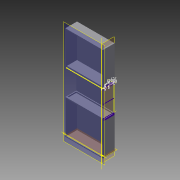
# Autodesk Inventor part: kontroller
Saved by Autodesk Inventor 2015 (Build 190159000, 159)
## iProperties
Created: 2015-12-13
Part Number: kontroller
Material: Generic
Document SubType Name: Modeling
Designer: abberik
Density: 1 g/cm^3
Appearance: Default
Author: abberik
Autodesk Inventor part; units mm, degrees
sketch "Sketch1" plane through (0, 0, 0) normal (0, 1, 0) x (-1, 0, 0)
  point P0 (0, 0)
sketch "Sketch2" plane through (0, 0, 0) normal (0, 1, 0) x (-1, 0, 0)
  point P0 (0, 0)
sketch "Sketch3" plane through (0, 0, 0) normal (0, 1, 0) x (-1, 0, 0)
  line L0 (93.3518, 235.1866) -> (-3.1482, 235.1866)
  line L1 (-3.1482, 235.1866) -> (-3.1482, -6.0634)
  line L2 (-3.1482, -6.0634) -> (93.3518, -6.0634)
  line L3 (93.3518, -6.0634) -> (93.3518, 235.1866)
  point P0 (0, 0)
  dimension "d0" = 241.25
  dimension "d1" = 96.5
  constraints: 8 end point, 2 parallel, 1 horizontal, 1 perpendicular
  measures "d0" distance of L2.end L0.start
  measures "d1" distance between parallel lines of L1 L3
extrude "Extrusion1" add sketch "Sketch3" along normal blind 30
sketch "Sketch4" plane through (0, 0, 0) normal (0, -1, 0) x (1, 0, 0)
  line L0 (-93.3518, -6.0634) -> (-93.3518, 235.1866) projected
  line L1 (-93.3518, 82.5616) -> (3.1482, 82.5616)
  line L2 (3.1482, 82.5616) -> (3.1482, 146.5616)
  line L3 (3.1482, 146.5616) -> (-93.3518, 146.5616)
  line L4 (-93.3518, 146.5616) -> (-93.3518, 82.5616)
  point P0 (0, 0)
  point P1 (-93.3518, 114.5616)
  point P2 (-93.3518, 114.5616)
  dimension "d4" = 64
  dimension "d5" = 0
  dimension "d6" = 96.5
  dimension "d7" = 0
  constraints: 8 end point, 2 midpoint, 2 parallel, 1 horizontal, 1 perpendicular
  measures "d4" distance between parallel lines of L3 L1
  measures "d5" distance of point (-93.352, 114.562) point (-93.352, 114.562)
  measures "d6" distance between parallel lines of L2 L4
  measures "d7" distance between parallel lines of L0 L4
extrude "Extrusion2" cut sketch "Sketch4" against normal blind 28
sketch "Sketch5" plane through (0, 0, 0) normal (0, -1, 0) x (1, 0, 0)
  line L0 (3.1482, 82.5616) -> (-93.3518, 82.5616) projected
  line L1 (-93.3518, -6.0634) -> (-93.3518, 82.5616) projected
  line L2 (3.1482, -6.0634) -> (-93.3518, -6.0634) projected
  line L3 (3.1482, 82.5616) -> (3.1482, -6.0634) projected
  line L4 (-93.3518, 146.5616) -> (3.1482, 146.5616) projected
  line L5 (3.1482, 235.1866) -> (3.1482, 146.5616) projected
  line L6 (-93.3518, 235.1866) -> (3.1482, 235.1866) projected
  line L7 (-93.3518, 146.5616) -> (-93.3518, 235.1866) projected
  line L8 (-91.3518, 80.5616) -> (1.1482, 80.5616)
  line L9 (1.1482, 80.5616) -> (1.1482, -4.0634)
  line L10 (1.1482, -4.0634) -> (-91.3518, -4.0634)
  line L11 (-91.3518, -4.0634) -> (-91.3518, 80.5616)
  line L12 (-91.3518, 233.1866) -> (1.1482, 233.1866)
  line L13 (1.1482, 233.1866) -> (1.1482, 148.5616)
  line L14 (1.1482, 148.5616) -> (-91.3518, 148.5616)
  line L15 (-91.3518, 148.5616) -> (-91.3518, 233.1866)
  point P0 (0, 0)
  dimension "d10" = 2
  dimension "d11" = 2
  constraints: 16 end point, 6 other
  measures "d10" distance between parallel lines of L1 L11
  measures "d11" distance between parallel lines of L7 L15
extrude "Extrusion3" cut sketch "Sketch5" against normal blind 28 contours L8 L9 L10 L11 | L12 L13 L14 L15
sketch "Sketch6" plane through (-93.3518, 0, 235.1866) normal (-1, 0, 0) x (0, 0, 1)
  point P0 (-235.1866, 0)
  point P1 (-196.9375, 14)
sketch "Sketch7" plane through (-91.3518, 0, 148.5616) normal (0, 0, 1) x (1, 0, 0)
  line L0 (92.5, 0) -> (0, 0) projected
  line L1 (92.5, 0) -> (92.5, 28) projected
  line L2 (92.5, 28) -> (0, 28) projected
  line L3 (0, 0) -> (0, 28) projected
  point P0 (91.3518, 0)
sketch "Sketch9" plane through (3.1482, 0, -6.0634) normal (1, 0, 0) x (0, 0, -1)
  line L0 (-152.625, 28) -> (-152.625, 26)
  line L1 (-152.625, 0) -> (-152.625, 28) projected
  line L2 (-152.625, 0) -> (-152.625, 4)
  line L3 (-152.625, 4) -> (-155.625, 4)
  line L4 (-155.625, 4) -> (-155.625, 26)
  line L5 (-155.625, 26) -> (-152.625, 26)
  line L6 (-152.625, 26) -> (-152.625, 4)
  line L7 (-88.625, 28) -> (-152.625, 28) projected
  line L8 (-120.625, 28) -> (-120.625, 0)
  line L9 (-88.625, 0) -> (-88.625, 28)
  line L10 (-88.625, 4) -> (-85.625, 4)
  line L11 (-85.625, 4) -> (-85.625, 26)
  line L12 (-85.625, 26) -> (-88.625, 26)
  line L13 (-88.625, 26) -> (-88.625, 4)
  line L14 (-152.625, 28) -> (-157.625, 28)
  line L15 (-157.625, 28) -> (-157.625, 2)
  line L16 (-157.625, 2) -> (-152.625, 2)
  line L17 (-88.625, 28) -> (-83.625, 28)
  line L18 (-83.625, 28) -> (-83.625, 2)
  line L19 (-83.625, 2) -> (-88.625, 2)
  line L20 (-152.625, 26) -> (-152.625, 28)
  line L21 (-154.625, 0) -> (-154.625, 28) projected
  line L22 (-152.625, 2) -> (-152.625, 4)
  line L23 (-152.625, 26) -> (-152.625, 4)
  line L24 (-88.625, 2) -> (-88.625, 4)
  line L25 (-88.625, 0) -> (-88.625, 28) projected
  line L26 (-88.625, 4) -> (-88.625, 26)
  line L27 (-88.625, 28) -> (-88.625, 26)
  point P0 (-6.0634, 0)
  dimension "d28" = 2
  dimension "d29" = 4
  dimension "d30" = 3
  dimension "d31" = 2
  dimension "d36" = 22
  dimension "d37" = 2
  dimension "d38" = 5
  constraints: 48 end point, 9 symmetric about line, 6 collinear, 5 perpendicular, 4 point on line, 1 midpoint, 1 parallel, 1 vertical, 2 other
  measures "d28" distance of L0.start L0.end
  measures "d29" distance of L1.start L2.end
  measures "d30" distance of L2.end L3.end
  measures "d31" distance between parallel lines of L4 L15
  measures "d36" distance of L3.end L4.end
  measures "d37" distance between parallel lines of L14 L5
  measures "d38" distance of L14.start L14.end
extrude "Extrusion5" add sketch "Sketch9" against normal up to surface (96.5 mm away) contours L17 L18 L19 L9 L10 L11 L12 | L0 L5 L21 L14 | L21 L5 L4 L3 L16 L15 L14 | L1 L16 L21 L3
extrude "Extrusion6" cut sketch "Sketch9" against normal blind 94.5 contours L1 L3 L21 L5 | L21 L3 L4 L5 | L12 L11 L10 L9
sketch "Sketch11" plane through (3.1482, 4, 149.5616) normal (0, 0, -1) x (-1, 0, 0)
  point P0 (3.1482, -4)
body "Solid1"
